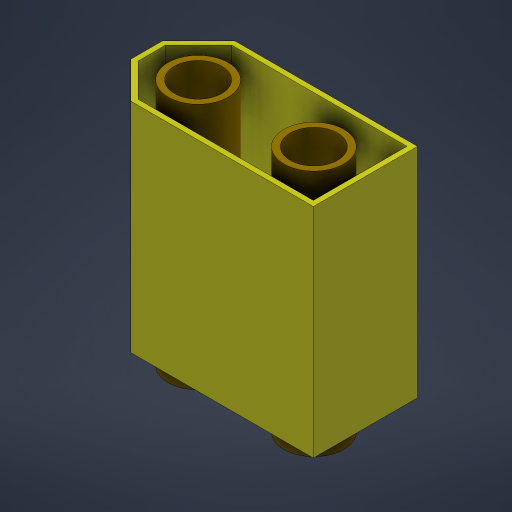
# Autodesk Inventor part: XT90NE-M
Saved by Autodesk Inventor 2023.5 (Build 275446000, 446)
## iProperties
Created: 2025-03-24
Part Number: XT90NE-M
Material: PC/ABS-Kunststoff
Document SubType Name: Modeling
Designer: David Lill
Density: 0.357273 g/cm^3
Appearance: Glatt - Gelb
Author: David Lill
Autodesk Inventor part; units mm, degrees
ref_plane "YZ Plane" through (0, 0, 0) normal (1, 0, 0) x (0, 1, 0)
ref_plane "XZ Plane" through (0, 0, 0) normal (0, 1, 0) x (-1, 0, 0)
ref_plane "XY Plane" through (0, 0, 0) normal (0, 0, 1) x (1, 0, 0)
sketch "Skizze1" plane through (0, 0, 0) normal (0, 0, 1) x (1, 0, 0)
  line L0 (0, 9.9) -> (0, 0)
  line L1 (0, 0) -> (-17.35, 0)
  line L2 (-17.35, 0) -> (-20.8, 3.45)
  line L3 (-20.8, 3.45) -> (-20.8, 6.45)
  line L4 (-20.8, 6.45) -> (-17.35, 9.9)
  line L5 (-17.35, 9.9) -> (0, 9.9)
  circle A0 centre (-15.9, 4.95) radius 2.85
  circle A1 centre (-4.9, 4.95) radius 2.85
  line L6 (-0.5, 9.4) -> (-0.5, 0.5)
  line L7 (-0.5, 0.5) -> (-17.1429, 0.5)
  line L8 (-17.1429, 0.5) -> (-20.3, 3.6571)
  line L9 (-20.3, 3.6571) -> (-20.3, 6.2429)
  line L10 (-20.3, 6.2429) -> (-17.1429, 9.4)
  line L11 (-17.1429, 9.4) -> (-0.5, 9.4)
  circle A2 centre (-15.9, 4.95) radius 2.25
  circle A3 centre (-4.9, 4.95) radius 2.25
  point P0 (0, 4.95)
  dimension "d2" = 20.8
  dimension "d4" = 45
  dimension "d5" = 9.9
  dimension "d6" = 3
  dimension "d8" = 5.7
  dimension "d9" = 11
  dimension "d11" = 4.9
  dimension "d12" = 0.5
  dimension "d13" = 4.5
  constraints: 24 end point, 4 centre point, 4 parallel, 3 coincident, 3 perpendicular, 2 equal radius, 2 horizontal alignment, 1 midpoint, 1 vertical, 1 vertical alignment, 5 other
  measures "d2" distance between parallel lines of L3 L0
  measures "d4" angle of L4 L5
  measures "d5" distance of L0.start L0.end
  measures "d6" distance of L2.end L3.end
  measures "d8" diameter of A0
  measures "d9" distance of A1.centre A0.centre
  measures "d11" distance from line of L0 A1.centre
  measures "d12" distance between parallel lines of L5 L11
  measures "d13" diameter of A2
extrude "Extrusion1" add sketch "Skizze1" against normal blind 20.7 contours L0 L1 L2 L3 L4 L5 | A0 | A1 | L6 L7 L8 L9 L10 L11 | A2 | A3
extrude "Extrusion2" add sketch "Skizze1" against normal blind 23.5 contours A0 | A1 | A2 | A3
extrude "Extrusion3" cut sketch "Skizze1" against normal blind 15 contours L6 L7 L8 L9 L10 L11 | A2 | A3
equation "\"d11\" = -0.5 * d9 + 0.5 * d2"
